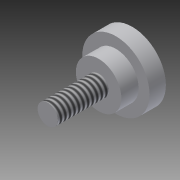
# Autodesk Inventor part: fastener_screw
Saved by Autodesk Inventor 2014 (Build 180170000, 170)
## iProperties
Created: 2014-03-24
Part Number: fastener_screw
Material: Generic
Document SubType Name: Modeling
Designer: stephenholtz
Density: 1 g/cm^3
Appearance: Default
Author: stephenholtz
Autodesk Inventor part; units mm, degrees
ref_plane "YZ Plane" through (0, 0, 0) normal (1, 0, 0) x (0, 1, 0)
ref_plane "XZ Plane" through (0, 0, 0) normal (0, 1, 0) x (-1, 0, 0)
ref_plane "XY Plane" through (0, 0, 0) normal (0, 0, 1) x (1, 0, 0)
sketch "Sketch1" plane through (0, 0, 0) normal (0, 0, 1) x (1, 0, 0)
  circle A0 centre (0, 0) radius 4.699
  dimension "head_dia" = 9.398
  constraints: 1 centre point, 1 coincident
  measures "head_dia" diameter of A0
extrude "Extrusion1" add sketch "Sketch1" along normal blind 2.286
sketch "Sketch2" plane through (0, 0, 2.286) normal (0, 0, 1) x (1, 0, 0)
  circle A0 centre (0, 0) radius 3.175
  dimension "d5" = 6.35
  constraints: 1 centre point, 1 coincident
  measures "d5" diameter of A0
extrude "Extrusion2" add sketch "Sketch2" along normal blind 2.413
sketch "Sketch3" plane through (0, 0, 4.699) normal (0, 0, 1) x (1, 0, 0)
  circle A0 centre (0, 0) radius 1.4224
  dimension "d8" = 2.8448
  constraints: 1 centre point, 1 coincident
  measures "d8" diameter of A0
extrude "Extrusion3" add sketch "Sketch3" along normal blind 7.112
thread "Thread1" size "4-40 UNC" class "2A" standard "ANSI Unified Screw Threads" full length
body "Solid1"
